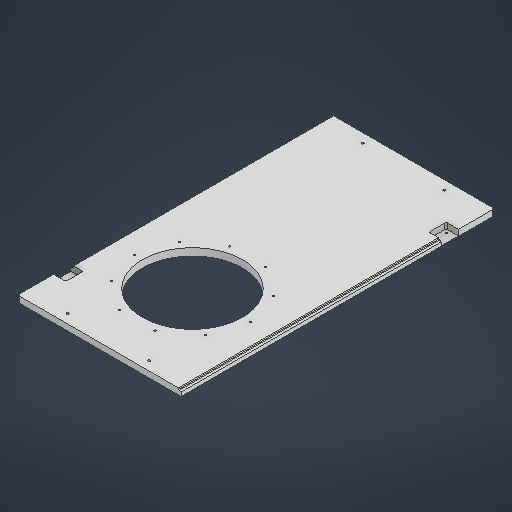
# Autodesk Inventor part: Updated Cover
Saved by Autodesk Inventor 2025 (Build 290162000, 162)
## iProperties
Created: 2024-04-25
Part Number: Updated Cover
Material: Generic
Document SubType Name: Modeling
Designer: Thienan Hoang
Density: 1 g/cm^3
Appearance: Default
Author: Thienan Hoang
Autodesk Inventor part; units mm, degrees
ref_plane "YZ Plane" through (0, 0, 0) normal (1, 0, 0) x (0, 1, 0)
sketch "Sketch1" plane through (0, 0, 0) normal (0, 1, 0) x (-1, 0, 0)
  line L0 (180, 345) -> (-180, 345)
  line L1 (-180, 345) -> (-180, -345)
  line L2 (-180, -345) -> (180, -345)
  line L3 (180, -345) -> (180, 345)
  line L4 (180, 345) -> (-180, -345) construction
  line L5 (-180, 345) -> (180, -345) construction
  point P0 (0, 0)
  dimension "d0" = 360
  dimension "d1" = 690
  constraints: 12 end point, 2 midpoint, 2 parallel, 1 horizontal, 1 perpendicular
  measures "d0" distance of L2.end L1.end
  measures "d1" distance of L1.end L0.end
extrude "Extrusion1" add sketch "Sketch1" along normal blind 15.875
sketch "Sketch2" plane through (0, 15.875, 0) normal (0, 1, 0) x (1, 0, 0)
  circle A0 centre (0, -140) radius 110
  line L0 (-180, -345) -> (180, -345) projected
  circle A1 centre (0, -140) radius 135
  point P0 (0, 0)
  dimension "d4" = 205
  dimension "d5" = 220
  dimension "d8" = 270
  constraints: 2 centre point, 1 coincident
  measures "d4" distance from line of A0.centre L0
  measures "d5" diameter of A0
  measures "d8" diameter of A1
extrude "Extrusion2" cut sketch "Sketch2" against normal through all contours A0
ref_plane "Work Plane1" through (0, 0, 150) normal (0, 0, 1) x (1, 0, 0)
sketch "Sketch6" plane through (0, 15.875, 0) normal (0, 1, 0) x (1, 0, 0)
  line L0 (89.6938, -325) -> (-89.6938, -325)
  line L1 (-89.6938, -325) -> (-89.6938, 325)
  line L2 (-89.6938, 325) -> (89.6938, 325)
  line L3 (89.6938, 325) -> (89.6938, -325)
  line L4 (89.6938, -325) -> (-89.6938, 325) construction
  line L5 (-89.6938, -325) -> (89.6938, 325) construction
  point P0 (0, 0)
  dimension "d55" = 179.3875
  dimension "d56" = 650
  constraints: 12 end point, 2 midpoint, 2 parallel, 1 horizontal, 1 perpendicular
  measures "d55" distance of L1.end L2.end
  measures "d56" distance of L0.end L1.end
hole "Hole3" at (89.6938, 15.875, 325) at (-89.6938, 15.875, 325) at (-89.6938, 15.875, -325) at (89.6938, 15.875, -325) direction (0, -1, 0) diameter 4.917 depth 5 tip angle 118 thread size "M6x1" class "6H" standard "ANSI Metric M Profile"
sketch "Sketch7" plane through (0, 15.875, 0) normal (0, 1, 0) x (1, 0, 0)
  circle A0 centre (0, -140) radius 110 projected
  circle A1 centre (0, -140) radius 131.5
  circle A2 centre (0, -140) radius 135
  point P0 (0, 0)
  dimension "d64" = 263
  dimension "d65" = 270
  constraints: 2 centre point, 2 coincident
  measures "d64" diameter of A1
  measures "d65" diameter of A2
ref_plane "Work Plane2" through (0, 15.875, 140) normal (0, 1, 0) x (1, 0, 0)
sketch "Sketch8" plane through (0, 15.875, 140) normal (0, 1, 0) x (1, 0, 0)
  circle A0 centre (0, 0) radius 131.5 projected
  circle A1 centre (0, 0) radius 127.5
  circle A2 centre (127.5, 0) radius 2
  circle A3 centre (103.1497, 74.9426) radius 2
  circle A4 centre (39.3997, 121.2597) radius 2
  circle A5 centre (-39.3997, 121.2597) radius 2
  circle A6 centre (-103.1497, 74.9426) radius 2
  circle A7 centre (-127.5, 0) radius 2
  circle A8 centre (-103.1497, -74.9426) radius 2
  circle A9 centre (-39.3997, -121.2597) radius 2
  circle A10 centre (39.3997, -121.2597) radius 2
  circle A11 centre (103.1497, -74.9426) radius 2
  point P0 (0, 140)
  dimension "d68" = 255
  dimension "d69" = 4
  dimension "d72" = 360
  constraints: 10 centre point, 1 coincident, 1 horizontal alignment, 23 other
  measures "d69" diameter of A2
hole "Hole4" at (127.5, 15.875, 140) at (103.1497, 15.875, 214.9426) at (39.3997, 15.875, 261.2597) at (-39.3997, 15.875, 261.2597) at (-103.1497, 15.875, 214.9426) at (-127.5, 15.875, 140) at (-103.1497, 15.875, 65.0574) at (-39.3997, 15.875, 18.7403) at (39.3997, 15.875, 18.7403) at (103.1497, 15.875, 65.0574) direction (0, -1, 0) diameter 4.134 depth 10 tip angle 118 thread size "M5x0.8" class "6H" standard "ANSI Metric M Profile"
sketch "Sketch9" plane through (0, 15.875, 0) normal (0, 1, 0) x (1, 0, 0)
  line L0 (180, -345) -> (180, 345) projected
  line L1 (180, 266) -> (156, 266)
  line L2 (153, 263) -> (153, 231)
  line L3 (156, 228) -> (180, 228)
  line L4 (180, 228) -> (180, 266)
  line L5 (-180, 345) -> (-180, -345) projected
  line L6 (-180, -266) -> (-156, -266)
  line L7 (-153, -263) -> (-153, -231)
  line L8 (-156, -228) -> (-180, -228)
  line L9 (-180, -228) -> (-180, -266)
  line L10 (180, 345) -> (-180, 345) projected
  line L11 (-180, -345) -> (180, -345) projected
  arc A0 (153, 231) -> (156, 228) centre (156, 231) ccw
  arc A1 (156, 266) -> (153, 263) centre (156, 263) ccw
  arc A2 (-156, -266) -> (-153, -263) centre (-156, -263) ccw
  arc A3 (-153, -231) -> (-156, -228) centre (-156, -231) ccw
  point P0 (0, 0)
  point P1 (153, 228)
  point P2 (153, 266)
  point P3 (-153, -228)
  point P4 (-153, -266)
  dimension "d82" = 27
  dimension "d83" = 27
  dimension "d84" = 38
  dimension "d85" = 38
  dimension "d86" = 79
  dimension "d87" = 79
  dimension "d95" = 3
  dimension "d96" = 3
  constraints: 16 end point, 10 point on line, 8 point on circle, 8 tangent, 4 centre point, 4 parallel, 2 equal radius, 2 horizontal, 2 perpendicular
  measures "d82" distance of L1.start point (153, 266)
  measures "d83" distance of point (-153, -228) L8.end
  measures "d84" distance of point (-153, -266) point (-153, -228)
  measures "d85" distance of point (153, 266) point (153, 228)
  measures "d86" distance between parallel lines of L10 L1
  measures "d87" distance between parallel lines of L11 L6
  measures "d95" radius of A0
  measures "d96" radius of A1
fillet "Fillet2" radius 5 2 edges at (180, 7.9375, -345) (-180, 7.9375, 345)
extrude "Extrusion7" cut sketch "Sketch9" against normal blind 12.575 contours L3 A0 L2 A1 L1 L0 | L5 L8 A3 L7 A2 L6
sketch "Sketch10" plane through (0, 15.875, 0) normal (0, 1, 0) x (1, 0, 0)
  line L0 (-180, -266) -> (-180, -228) projected
  line L1 (175, 345) -> (-180, 345) projected
  line L2 (-180, -228) -> (-174, -228)
  line L3 (-174, -228) -> (-174, 345)
  line L4 (-174, 345) -> (-180, 345)
  line L5 (-180, 345) -> (-180, -228)
  line L6 (180, 228) -> (156, 228) projected
  line L7 (-175, -345) -> (180, -345) projected
  line L8 (180, 228) -> (174, 228)
  line L9 (174, 228) -> (174, -345)
  line L10 (174, -345) -> (180, -345)
  line L11 (180, -345) -> (180, 228)
  point P0 (0, 0)
  point P1 (180, -345)
  dimension "d99" = 6
  dimension "d100" = 6
  constraints: 16 end point, 4 parallel, 2 horizontal, 2 perpendicular, 2 point on line
  measures "d99" distance of L4.end L3.end
  measures "d100" distance of L10.end L9.end
extrude "Extrusion8" cut sketch "Sketch10" against normal blind 3.1
chamfer "Chamfer3" distance 2 distance2 3.5 1 edges at (180, 12.775, 58.5) measured on face at (180, 5.3583, 154)
chamfer "Chamfer4" distance 3.5 distance2 2 1 edges at (-180, 12.775, -58.5) measured on face at (-180, 5.3583, -154)
sketch "Sketch11" plane through (0, 3.3, 0) normal (0, 1, 0) x (1, 0, 0)
  circle A0 centre (-161, -236) radius 1.65
  circle A1 centre (-161, -258) radius 1.65
  circle A2 centre (161, 258) radius 1.65
  circle A3 centre (161, 236) radius 1.65
  line L0 (-180, -266) -> (-180, -228) projected
  line L1 (-156, -266) -> (-180, -266) projected
  line L2 (174, 228) -> (156, 228) projected
  line L3 (180, 266) -> (180, 228) projected
  point P0 (0, 0)
  dimension "d109" = 19
  dimension "d110" = 8
  dimension "d111" = 22
  dimension "d112" = 19
  dimension "d113" = 3.3
  dimension "d114" = 3.3
  dimension "d115" = 3.3
  dimension "d116" = 3.3
  dimension "d118" = 8
  dimension "d119" = 22
  dimension "d120" = 19
  dimension "d121" = 19
  constraints: 4 centre point
  measures "d109" distance from line of L0 A1.centre
  measures "d110" distance from line of L1 A1.centre
  measures "d111" distance of A1.centre A0.centre
  measures "d112" distance from line of L0 A0.centre
  measures "d113" diameter of A0
  measures "d114" diameter of A1
  measures "d115" diameter of A3
  measures "d116" diameter of A2
  measures "d118" distance from line of L2 A3.centre
  measures "d119" distance of A3.centre A2.centre
  measures "d120" distance from line of L3 A2.centre
  measures "d121" distance from line of L3 A3.centre
hole "Hole5" at (-161, 3.3, 258) at (-161, 3.3, 236) at (161, 3.3, -236) at (161, 3.3, -258) direction (0, -1, 0) diameter 3.242 end through all thread size "M4x0.7" class "6H" standard "ANSI Metric M Profile"
chamfer "Chamfer5" distance 0.35 angle 45 4 edges at (-161, 3.3, 256.379) (-161, 3.3, 234.379) (161, 3.3, -259.621) (161, 3.3, -237.621)
chamfer "Chamfer6" distance 2.5 angle 45 3 edges at (178.5355, 0, -343.5355) (-2.5, 0, -345) (180, 0, 2.5)
chamfer "Chamfer7" distance 2.5 angle 45 3 edges at (-178.5355, 0, 343.5355) (1.25, 0, 345) (-180, 0, -1.25)
body "Solid1"
